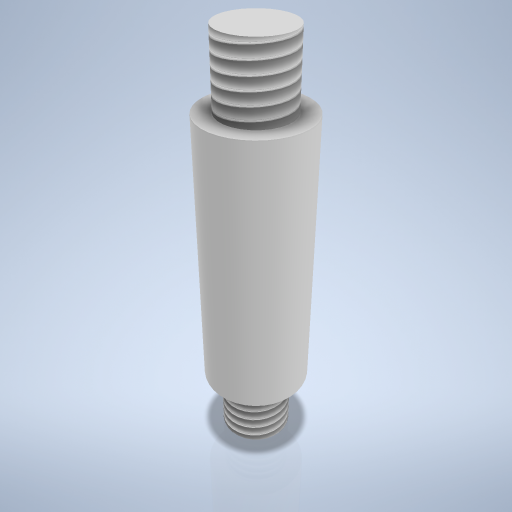
# Autodesk Inventor part: welle_verbindung
Saved by Autodesk Inventor 2024.2 (Build 282272000, 272)
## iProperties
Created: 2024-05-05
Part Number: welle_verbindung
Material: Generisch
Document SubType Name: Modeling
Designer: Fabri
Density: 1 g/cm^3
Appearance: Vorgabe
Author: Fabri
Autodesk Inventor part; units mm, degrees
ref_plane "YZ Plane" through (0, 0, 0) normal (1, 0, 0) x (0, 1, 0)
ref_plane "XZ Plane" through (0, 0, 0) normal (0, 1, 0) x (-1, 0, 0)
ref_plane "XY Plane" through (0, 0, 0) normal (0, 0, 1) x (1, 0, 0)
sketch "Skizze1" plane through (0, 0, 0) normal (0, 1, 0) x (-1, 0, 0)
  line L0 (0, 18) -> (3, 18)
  line L1 (3, 18) -> (3, 12)
  line L2 (3, 12) -> (4.5, 12)
  line L3 (4.5, 12) -> (4.5, -12)
  line L4 (4.5, -12) -> (3, -12)
  line L5 (3, -12) -> (3, -18)
  line L6 (3, -18) -> (0, -18)
  line L7 (0, -18) -> (0, 18)
  point P0 (0, 0)
  point P1 (0, 0)
  dimension "d0" = 6
  dimension "d1" = 6
  dimension "d2" = 24
  dimension "d3" = 9
  dimension "d4" = 6
  constraints: 16 end point, 6 perpendicular, 2 point on line, 1 coincident, 1 horizontal, 1 midpoint
  measures "d0" distance between parallel lines of L2 L0
  measures "d1" distance between parallel lines of L6 L4
  measures "d2" distance of L2.end L3.end
  measures "d3" diameter of L3 L7
  measures "d4" diameter of L5 L7
revolve "Umdrehung1" add sketch "Skizze1" angle 360 about axis through (0, 0, -18) along (0, 0, 1)
thread "Gewinde1" size "M6x1" class "6g" standard "ISO Metric profile" length 18
thread "Gewinde2" size "M6x1" class "6g" standard "ISO Metric profile" length 18
